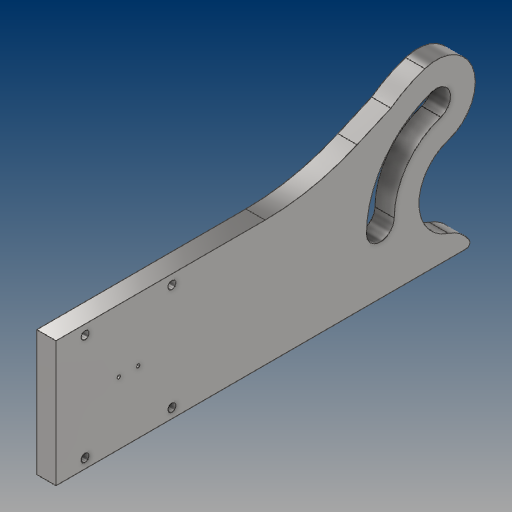
# Autodesk Inventor part: 16_Khau_hai
Saved by Autodesk Inventor 2021 (Build 250183000, 183)
## iProperties
Created: 2024-04-05
Part Number: 16_Khau_hai
Material: Stainless Steel, Austenitic
Document SubType Name: Modeling
Designer: Admin
Density: 8 g/cm^3
Appearance: Semi-Polished
Author: Admin
Autodesk Inventor part; units mm, degrees
ref_plane "YZ Plane" through (0, 0, 0) normal (1, 0, 0) x (0, 1, 0)
ref_plane "XZ Plane" through (0, 0, 0) normal (0, 1, 0) x (-1, 0, 0)
ref_plane "XY Plane" through (0, 0, 0) normal (0, 0, 1) x (1, 0, 0)
sketch "Sketch1" plane through (0, 0, 0) normal (1, 0, 0) x (0, 1, 0)
  line L0 (-27.5, 22.5) -> (27.5, 22.5)
  line L1 (27.5, 22.5) -> (27.5, -22.5)
  line L2 (27.5, -22.5) -> (-27.5, -22.5)
  line L3 (-27.5, -22.5) -> (-27.5, 22.5)
  line L4 (-27.5, 22.5) -> (27.5, -22.5) construction
  line L5 (27.5, 22.5) -> (-27.5, -22.5) construction
  line L6 (32.5, 37.5) -> (-32.5, 37.5)
  line L7 (-32.5, 37.5) -> (-32.5, -162.5)
  line L8 (-32.5, -162.5) -> (32.5, -162.5)
  line L9 (32.5, -162.5) -> (32.5, 37.5)
  line L10 (0, 0) -> (0, -107.0279) construction
  dimension "d0" = 45
  dimension "d1" = 55
  dimension "d2" = 65
  dimension "d3" = 200
  dimension "d4" = 15
  constraints: 22 end point, 4 parallel, 2 horizontal, 2 midpoint, 2 perpendicular, 1 vertical, 1 other
  measures "d0" distance of L0.end L1.end
  measures "d1" distance of L1.end L2.end
  measures "d2" distance of L6.start L6.end
  measures "d3" distance of L8.end L6.start
  measures "d4" distance between parallel lines of L6 L0
extrude "Extrusion1" add sketch "Sketch1" along normal mid plane 10 contours L0 L1 L2 L3 | L9 L8 L7 L6
hole "Hole1" at (0, 27.5, 22.5) at (0, -27.5, 22.5) at (0, -27.5, -22.5) at (0, 27.5, -22.5) direction (-1, 0, 0) diameter 4.2 end through all both
sketch "Sketch3" plane through (5, 0, 0) normal (1, 0, 0) x (0, 0, -1)
  circle A0 centre (22.5, -27.5) radius 2.1 projected
  circle A1 centre (-22.5, 27.5) radius 2.1 projected
  circle A2 centre (-22.5, -27.5) radius 2.1 projected
  circle A3 centre (22.5, 27.5) radius 2.1 projected
  line L0 (-37.5, -32.5) -> (162.5, -32.5) projected
  line L1 (162.5, -32.5) -> (162.5, 32.5) projected
  line L2 (162.5, 32.5) -> (-37.5, 32.5) projected
  line L3 (-37.5, 32.5) -> (-37.5, -32.5) projected
  line L4 (162.5, 0) -> (-37.5, 0) construction
  line L5 (-37.5, 32.5) -> (-37.5, -32.5) projected
  line L6 (162.5, -32.5) -> (162.5, 32.5) projected
  arc A4 (159.6938, 40) -> (159.6938, -40) centre (172.5, 0) ccw construction
  arc A5 (153.5955, 59.0476) -> (153.5955, -59.0476) centre (172.5, 0) ccw
  arc A6 (165.792, 20.9524) -> (165.792, -20.9524) centre (172.5, 0) ccw
  arc A7 (165.792, 20.9524) -> (153.5955, 59.0476) centre (159.6938, 40) ccw
  arc A8 (153.5955, -59.0476) -> (165.792, -20.9524) centre (159.6938, -40) ccw
  arc A9 (157.4984, 46.8571) -> (157.4984, -46.8571) centre (172.5, 0) ccw
  arc A10 (157.4984, -46.8571) -> (161.8891, -33.1429) centre (159.6938, -40) ccw
  arc A11 (161.8891, 33.1429) -> (161.8891, -33.1429) centre (172.5, 0) ccw
  arc A12 (161.8891, 33.1429) -> (157.4984, 46.8571) centre (159.6938, 40) ccw
  circle A13 centre (130.5, 0) radius 7.2
  point P0 (0, 0)
  point P1 (162.5, 0)
  point P2 (135.5623, -32.5)
  point P3 (119.7009, -32.5)
  point P4 (113.3868, -25)
  point P5 (160.0585, -32.5)
  point P6 (160.0585, 32.5)
  point P7 (113.3868, 25)
  point P8 (119.7009, 32.5)
  point P9 (135.5623, 32.5)
  point P10 (116.802, 25)
  point P11 (116.802, -25)
  point P12 (123.3, 0)
  point P13 (137.7, 0)
  point P14 (162.5, -19.5959)
  point P15 (162.5, 19.5959)
  dimension "d27" = 42
  dimension "d28" = 20
  dimension "d29" = 10
  dimension "d30" = 80
  dimension "d32" = 7.2
  constraints: 19 point on circle, 10 centre point, 4 tangent, 3 midpoint, 2 end point, 1 equal radius, 4 other
  measures "d27" radius of A4
  measures "d28" radius of A7
  measures "d29" distance from line of L1 A4.centre
  measures "d30" distance of A4.end A4.start
  measures "d32" radius of A12
extrude "Extrusion2" add sketch "Sketch3" against normal blind 10 contours A5 L2 A9 L0 | L0 A9 A10 A11 L1 A6 A8 A5 | A9 A13 A11 L0 | L0 A11 A10 A9 | A5 A7 A6 L1 L2 A11 A12 A9 | A11 L2 L1 A6 L0 | A9 L2 A11 A13 | A13 | A9 A12 A11 L2
extrude "Extrusion3" cut sketch "Sketch3" against normal blind 85 contours A9 L2 A11 A13 | A13 | A9 A12 A11 L2
extrude "Extrusion4" cut sketch "Sketch3" against normal blind 85 contours A6 L1
chamfer "Chamfer1" distance 24 angle 45 2 edges at (0, 32.5, -119.7009) (0, -32.5, -119.7009)
fillet "Fillet1" radius 119 2 edges at (0, 32.5, -95.7009) (0, -32.5, -95.7009)
sketch "Sketch4" plane through (5, 0, 0) normal (1, 0, 0) x (0, 0, -1)
  arc A0 (118.4927, -42.4637) -> (70.8263, -32.5) centre (70.8263, -151.5) ccw projected
  line L0 (70.8263, -32.5) -> (178.2342, -32.5)
  arc A1 (153.5955, -59.0476) -> (165.792, -20.9524) centre (159.6938, -40) ccw projected
  arc A2 (135.9994, -50.1169) -> (153.5955, -59.0476) centre (172.5, 0) ccw projected
  line L1 (135.9994, -50.1169) -> (118.4927, -42.4637) projected
  point P0 (0, 0)
  constraints: 2 end point, 1 horizontal, 1 point on circle
extrude "Extrusion5" cut sketch "Sketch4" against normal blind 36.25
fillet "Fillet2" radius 2 1 edges at (0, -32.5, -178.2342)
sketch "Sketch5" plane through (5, 0, 0) normal (1, 0, 0) x (0, 0, -1)
  line L0 (0, 0) -> (0, 9.6714)
  line L1 (-5, 0) -> (5, 0)
  dimension "d46" = 10
  constraints: 4 end point, 1 horizontal, 1 symmetric about line, 1 vertical
  measures "d46" distance of L1.start L1.end
hole "Hole3" at (5, 0, -5) at (5, 0, 5) direction (-1, 0, 0) diameter 1.8 end through all
body "Solid1"
